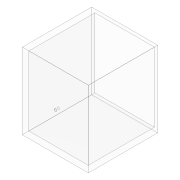
# Autodesk Inventor part: Deckel_Koch_final
Saved by Autodesk Inventor 2020 (Build 240168000, 168)
## iProperties
Created: 2022-02-08
Part Number: Deckel_Koch_final
Material: PMMA-Kunststoff
Document SubType Name: Modeling
Designer: Julian Uhl
Density: 1.188 g/cm^3
Appearance: Polycarbonat - klar
Author: Julian Uhl
Autodesk Inventor part; units mm, degrees
ref_plane "YZ Plane" through (0, 0, 0) normal (1, 0, 0) x (0, 1, 0)
ref_plane "XZ Plane" through (0, 0, 0) normal (0, 1, 0) x (-1, 0, 0)
ref_plane "XY Plane" through (0, 0, 0) normal (0, 0, 1) x (1, 0, 0)
sketch "Skizze1" plane through (0, 0, 0) normal (0, 0, 1) x (1, 0, 0)
  line L0 (-20, 0) -> (120, 0) projected
  line L1 (0, -23) -> (0, 138) projected
  line L2 (0, 0) -> (100, 0)
  line L3 (100, 0) -> (100, 115)
  line L4 (100, 115) -> (0, 115)
  line L5 (0, 115) -> (0, 0)
  line L6 (5, 5) -> (95, 5)
  line L7 (95, 5) -> (95, 110)
  line L8 (95, 110) -> (5, 110)
  line L9 (5, 110) -> (5, 5)
  point P0 (0, 115)
  dimension "d0" = 5
  dimension "d1" = 5
  dimension "d2" = 5
  dimension "d3" = 5
  dimension "d4" = 90
  dimension "d5" = 105
  constraints: 16 end point, 4 parallel, 2 horizontal, 2 perpendicular
  measures "d0" distance between parallel lines of L4 L8
  measures "d1" distance between parallel lines of L1 L9
  measures "d2" distance between parallel lines of L0 L6
  measures "d3" distance between parallel lines of L3 L7
  measures "d4" distance between parallel lines of L9 L7
  measures "d5" distance between parallel lines of L8 L6
extrude "Extrusion1" add sketch "Skizze1" along normal blind 100
sketch "Skizze2" plane through (0, 0, 100) normal (0, 0, 1) x (1, 0, 0)
  line L0 (0, 115) -> (0, 0) projected
  line L1 (0, 0) -> (100, 0)
  line L2 (100, 0) -> (100, 115)
  line L3 (100, 115) -> (0, 115)
  line L4 (0, 115) -> (0, 0)
  constraints: 8 end point, 2 parallel, 1 horizontal, 1 perpendicular
extrude "Extrusion2" add sketch "Skizze2" along normal blind 5
sketch "Skizze3" plane through (0, 0, 105) normal (0, 0, 1) x (1, 0, 0)
  line L0 (100, 0) -> (100, 115) projected
  line L1 (100, 115) -> (0, 115) projected
  point P0 (0, 0)
  point P1 (50, 57.5)
  dimension "d10" = 50
  dimension "d11" = 57.5
  measures "d10" distance from line of point (50, 57.5) L0
  measures "d11" distance from line of L1 point (50, 57.5)
hole "Bohrung1" at (50, 57.5, 105) direction (0, 0, -1) diameter 3 end through all
fillet "Rundung1" radius 0.4 1 edges at (50, 59, 105)
